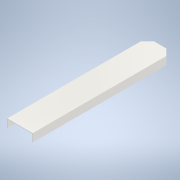
# Autodesk Inventor part: Horquilla_Cubierta
Saved by Autodesk Inventor 2022.1 (Build 261234000, 234)
## iProperties
Created: 2021-09-10
Part Number: Horquilla_Cubierta
Material: Genérico
Document SubType Name: Modeling
Designer: seb_0
Density: 1 g/cm^3
Appearance: Acero
Author: seb_0
Autodesk Inventor part; units mm, degrees
ref_plane "YZ Plane" through (0, 0, 0) normal (1, 0, 0) x (0, 1, 0)
ref_plane "XZ Plane" through (0, 0, 0) normal (0, 1, 0) x (-1, 0, 0)
ref_plane "XY Plane" through (0, 0, 0) normal (0, 0, 1) x (1, 0, 0)
sketch "Boceto1" plane through (0, 0, 0) normal (0, 1, 0) x (-1, 0, 0)
  line L0 (0, 0) -> (200, 0)
  line L1 (200, 0) -> (200, -1050)
  line L2 (150, -1100) -> (50, -1100)
  line L3 (0, -1050) -> (0, 0)
  line L4 (200, -1050) -> (150, -1100)
  line L5 (0, -1050) -> (50, -1100)
  circle A0 centre (100, -800) radius 15
  circle A1 centre (100, -300) radius 15
  point P0 (200, -1100)
  point P1 (0, -1100)
  dimension "d0" = 1100
  dimension "d1" = 200
  dimension "d2" = 50
  dimension "d3" = 50
  dimension "d4" = 50
  dimension "d5" = 50
  dimension "d11" = 30
  dimension "d12" = 30
  dimension "d13" = 300
  dimension "d14" = 500
  dimension "d15" = 100
  dimension "d16" = 100
  constraints: 12 end point, 4 point on line, 2 centre point, 2 parallel, 1 horizontal, 1 perpendicular
  measures "d0" distance of L0.end point (200, -1100)
  measures "d1" distance of point (200, -1100) point (0, -1100)
  measures "d2" distance of L1.end point (200, -1100)
  measures "d3" distance of L2.start point (200, -1100)
  measures "d4" distance of L3.start point (0, -1100)
  measures "d5" distance of L2.end point (0, -1100)
  measures "d11" diameter of A0
  measures "d12" diameter of A1
  measures "d13" distance from line of L0 A1.centre
  measures "d14" distance of A1.centre A0.centre
  measures "d15" distance from line of L1 A1.centre
  measures "d16" distance from line of L1 A0.centre
extrude "Extrusión1" add sketch "Boceto1" along normal blind 3 contours L0 L1 L4 L2 L5 L3 | A0 | A1
sketch "Boceto2" plane through (0, 0, 0) normal (0, -1, 0) x (1, 0, 0)
  line L0 (-50, -1100) -> (-150, -1100) projected
  line L1 (0, -1050) -> (-50, -1100) projected
  line L2 (0, 0) -> (0, -1050) projected
  line L3 (-200, 0) -> (0, 0) projected
  line L4 (-200, -1050) -> (-200, 0) projected
  line L5 (-150, -1100) -> (-200, -1050) projected
  line L6 (-2.5, -1048.9645) -> (-51.0355, -1097.5)
  line L7 (-51.0355, -1097.5) -> (-148.9645, -1097.5)
  line L8 (-148.9645, -1097.5) -> (-197.5, -1048.9645)
  line L9 (-197.5, -1048.9645) -> (-197.5, -2.5)
  line L10 (-197.5, -2.5) -> (-2.5, -2.5)
  line L11 (-2.5, -2.5) -> (-2.5, -1048.9645)
  line L12 (0, 0) -> (0, -1050) projected
  line L13 (0, -1050) -> (-3.5355, -1050)
  line L14 (-150, -1100) -> (-200, -1050) projected
  line L15 (-200, -1050) -> (-196.4645, -1050)
  line L16 (-197.5, -2.5) -> (-197.5, 0)
  line L17 (-200, 0) -> (0, 0) projected
  line L18 (-2.5, -2.5) -> (-2.5, 0)
  dimension "d8" = 2.5
  constraints: 20 end point, 5 point on line, 2 perpendicular, 1 horizontal, 5 other
  measures "d8" distance between parallel lines of L2 L11
extrude "Extrusión2" add sketch "Boceto2" along normal blind 60 contours L0 L5 L15 L8 L7 L6 L13 L1 | L13 L6 L11 L18 L3 L2 | L4 L3 L16 L9 L8 L15
equation "\"d3\" = d2"
equation "\"d4\" = d2"
equation "\"d5\" = d4"
